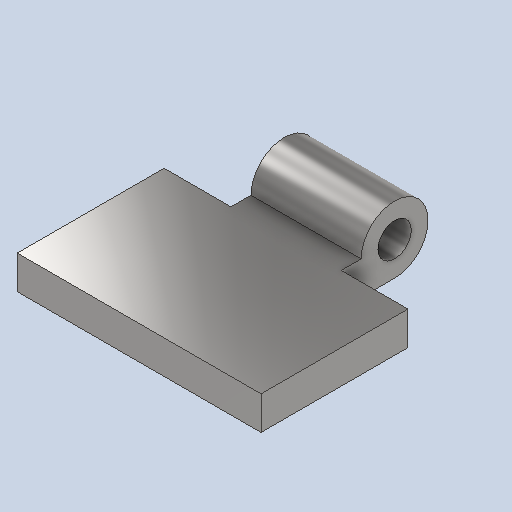
# Autodesk Inventor part: hinge 2
Saved by Autodesk Inventor 2022 (Build 260153000, 153)
## iProperties
Created: 2022-04-11
Part Number: hinge 2
Material: Stainless Steel
Document SubType Name: Modeling
Designer: MacBook
Density: 8 g/cm^3
Appearance: Semi-Polished
Author: MacBook
Autodesk Inventor part; units mm, degrees
ref_plane "YZ Plane" through (0, 0, 0) normal (1, 0, 0) x (0, 1, 0)
ref_plane "XZ Plane" through (0, 0, 0) normal (0, 1, 0) x (-1, 0, 0)
ref_plane "XY Plane" through (0, 0, 0) normal (0, 0, 1) x (1, 0, 0)
sketch "Sketch1" plane through (0, 0, 0) normal (0, 1, 0) x (-1, 0, 0)
  line L0 (-18.2565, -12.5) -> (18.2565, -12.5)
  line L1 (18.2565, -12.5) -> (18.2565, 12.5)
  line L2 (18.2565, 12.5) -> (-18.2565, 12.5)
  line L3 (-18.2565, 12.5) -> (-18.2565, -12.5)
  line L4 (-18.2565, -12.5) -> (18.2565, 12.5) construction
  line L5 (18.2565, -12.5) -> (-18.2565, 12.5) construction
  point P0 (0, 0)
  dimension "d0" = 36.513
  dimension "d1" = 25
  constraints: 12 end point, 2 midpoint, 2 parallel, 1 horizontal, 1 perpendicular
  measures "d0" distance between parallel lines of L3 L1
  measures "d1" distance between parallel lines of L0 L2
extrude "Extrusion1" add sketch "Sketch1" against normal blind 5
sketch "Sketch2" plane through (18.2565, 0, 12.5) normal (1, 0, 0) x (0, 0, -1)
  circle A0 centre (30, 0) radius 5
  line L0 (25, 0) -> (25, -5) projected
  line L1 (25, -5) -> (0, -5) projected
  line L2 (0, -5) -> (25, -5) projected
  line L3 (25, -5) -> (30, -5)
  line L4 (30, -5) -> (30, 0)
  line L5 (30, 0) -> (25, 0)
  line L6 (25, 0) -> (25, -5)
  point P0 (12.5, 0)
  dimension "d4" = 5
  dimension "d5" = 10
  dimension "d6" = 5
  constraints: 8 end point, 2 parallel, 1 centre point, 1 horizontal, 1 perpendicular
  measures "d4" distance from line of L0 L4.end
  measures "d5" diameter of A0
  measures "d6" distance from line of L1 L4.end
extrude "Extrusion2" add sketch "Sketch2" against normal blind 36.513
sketch "Sketch3" plane through (18.2565, -5, 12.5) normal (1, 0, 0) x (0, 0, -1)
  circle A0 centre (30, 5) radius 2.5
  line L0 (0, 0) -> (30, 0) projected
  line L1 (0, 5) -> (0, 0) projected
  point P0 (12.5, 5)
  dimension "d9" = 5
  dimension "d10" = 30
  dimension "d11" = 5
  constraints: 1 centre point
  measures "d9" distance from line of L0 A0.centre
  measures "d10" distance from line of L1 A0.centre
  measures "d11" diameter of A0
extrude "Extrusion3" cut sketch "Sketch3" against normal blind 36.513
sketch "Sketch4" plane through (0, -5, 0) normal (0, -1, 0) x (1, 0, 0)
  line L0 (18.2565, 12.5) -> (18.2565, -17.5) projected
  line L1 (18.2565, -9.5) -> (8.2565, -9.5)
  line L2 (8.2565, -9.5) -> (8.2565, -22.5)
  line L3 (8.2565, -22.5) -> (18.2565, -22.5)
  line L4 (18.2565, -22.5) -> (18.2565, -9.5)
  line L5 (-18.2565, -9.5) -> (-8.2565, -9.5)
  line L6 (-8.2565, -9.5) -> (-8.2565, -22.5)
  line L7 (-8.2565, -22.5) -> (-18.2565, -22.5)
  line L8 (-18.2565, -22.5) -> (-18.2565, -9.5)
  line L9 (18.2565, -17.5) -> (-18.2565, -17.5) projected
  line L10 (-18.2565, 12.5) -> (-18.2565, -17.5) projected
  point P0 (0, 0)
  point P1 (18.2565, -17.5)
  dimension "d14" = 5
  dimension "d15" = 16.513
  dimension "d16" = 0
  dimension "d17" = 10
  dimension "d18" = 13
  constraints: 16 end point, 4 parallel, 3 point on line, 2 horizontal, 2 perpendicular
  measures "d14" distance between parallel lines of L9 L3
  measures "d15" distance between parallel lines of L6 L2
  measures "d16" distance between parallel lines of L10 L8
  measures "d17" distance between parallel lines of L2 L0
  measures "d18" distance between parallel lines of L3 L1
extrude "Extrusion4" cut sketch "Sketch4" against normal blind 36.513
body "Solid1"
